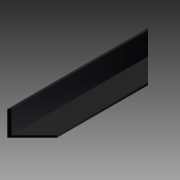
# Autodesk Inventor part: angle template al-6061 1x1x0.125
Saved by Autodesk Inventor 2012 (Build 160160000, 160)
## iProperties
Created: 2011-11-26
Part Number: angle template al-6061 1x1x0.125
Material: Aluminum-6061
Document SubType Name: Modeling
Designer: Antonella
Mass: 249.8 g
Surface Area: 622.378 cm^2
Volume: 92.1772 cm^3
Density: 2.71 g/cm^3
Author: Antonella
Autodesk Inventor part; units mm, degrees
ref_plane "YZ Plane" through (0, 0, 0) normal (1, 0, 0) x (0, 1, 0)
ref_plane "XZ Plane" through (0, 0, 0) normal (0, 1, 0) x (-1, 0, 0)
ref_plane "XY Plane" through (0, 0, 0) normal (0, 0, 1) x (1, 0, 0)
sketch "Sketch1" plane through (0, 0, 0) normal (0, 0, 1) x (1, 0, 0)
  line L0 (-26.67, 0) -> (26.67, 0) projected
  line L1 (0, -26.67) -> (0, 26.67) projected
  line L2 (-19.05, 19.05) -> (-19.05, -19.05)
  line L3 (-19.05, -19.05) -> (19.05, -19.05)
  line L4 (19.05, -15.875) -> (-15.875, -15.875)
  line L5 (-15.875, -15.875) -> (-15.875, 19.05)
  line L6 (-19.05, 19.05) -> (-15.875, 19.05)
  line L7 (19.05, -19.05) -> (19.05, -15.875)
  point P0 (0, 0)
  point P1 (-19.05, 0)
  point P2 (0, -19.05)
  dimension "d0" = 38.1
  dimension "d1" = 3.175
  constraints: 12 end point, 5 perpendicular, 2 midpoint, 1 horizontal alignment, 1 parallel, 1 vertical alignment, 1 other
  measures "d0" distance of L2.start L2.end
  measures "d1" distance between parallel lines of L4 L3
extrude "Extrusion1" add sketch "Sketch1" along normal mid plane 215.9 contours L2 L6 L5 L0 | L0 L5 L4 L1 L3 L2 | L1 L4 L7 L3
sketch "Sketch2" plane through (-15.875, -15.875, 107.95) normal (0, 1, 0) x (1, 0, 0)
  line L0 (0, 0) -> (34.925, 0) projected
  line L1 (34.925, 215.9) -> (34.925, 0) projected
  line L2 (0, 215.9) -> (0, 0) projected
  line L3 (-3.175, 0) -> (-3.175, 215.9) projected
  line L4 (-3.175, 0) -> (34.925, 38.1)
  line L5 (34.925, 107.95) -> (0, 107.95) construction
  line L6 (-3.175, 215.9) -> (34.925, 177.8)
  line L7 (-3.175, 0) -> (34.925, 0)
  line L8 (34.925, 0) -> (34.925, 38.1)
  line L9 (-3.175, 215.9) -> (34.925, 215.9)
  line L10 (34.925, 215.9) -> (34.925, 177.8)
  point P0 (15.875, 107.95)
  dimension "d4" = 45
  constraints: 14 end point, 2 collinear, 2 midpoint, 1 perpendicular, 1 point on line, 1 symmetric about line
  measures "d4" angle of L4 L0
extrude "Extrusion2" cut sketch "Sketch2" along normal through all both and the other way through all contours L2 L4 L1 L0 | L7 L4 L2 | L6 L9 L2 | L2 L9 L1 L6
body "Solid1"
